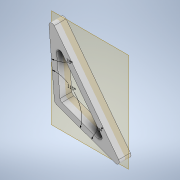
# Autodesk Inventor part: stopForSaltChute
Saved by Autodesk Inventor 2021.1 (Build 251245000, 245)
## iProperties
Created: 2020-09-07
Part Number: stopForSaltChute
Material: Generic
Document SubType Name: Modeling
Designer: robst
Density: 1 g/cm^3
Appearance: Default
Author: robst
Autodesk Inventor part; units mm, degrees
ref_plane "YZ Plane" through (0, 0, 0) normal (1, 0, 0) x (0, 1, 0)
ref_plane "XZ Plane" through (0, 0, 0) normal (0, 1, 0) x (-1, 0, 0)
sketch "Sketch1" plane through (0, 0, 0) normal (0, 0, 1) x (1, 0, 0)
  line L0 (0, 0) -> (-10.4993, 120.0076)
  line L1 (-10.4993, 120.0076) -> (113.201, -41.2018)
  line L2 (113.201, -41.2018) -> (0, 0)
  dimension "d23" = 115
  dimension "d24" = 203.2
  dimension "d31" = 32.5
  constraints: 6 end point
  measures "d23" angle of L2 L0
  measures "d24" distance of L0.end L1.end
  measures "d31" angle of L1 L2
extrude "Extrusion1" add sketch "Sketch1" along normal mid plane 19.05
sketch "Sketch2" plane through (0, 0, 0) normal (0, 0, 1) x (1, 0, 0)
  line L0 (8.9599, 6.8752) -> (1.8376, 88.2833)
  line L1 (1.8376, 88.2833) -> (85.7507, -21.0744)
  line L2 (85.7507, -21.0744) -> (8.9599, 6.8752)
  line L3 (0, 0) -> (-10.4993, 120.0076) projected
  line L4 (-10.4993, 120.0076) -> (113.201, -41.2018) projected
  line L5 (113.201, -41.2018) -> (0, 0) projected
  dimension "d4" = 9.525
  dimension "d5" = 9.525
  dimension "d6" = 9.525
  constraints: 6 end point, 3 parallel, 1 equal length, 1 other
  measures "d4" distance between parallel lines of L0 L3
  measures "d5" distance between parallel lines of L1 L4
  measures "d6" distance between parallel lines of L2 L5
extrude "Extrusion2" cut sketch "Sketch2" against normal through all both and the other way through all contours L0 L1 L2
fillet "Fillet1" radius 4.7625 3 edges at (-10.4993, 120.0076, 0) (0, 0, 0) (113.201, -41.2018, 0)
fillet "Fillet2" radius 4.7625 3 edges at (1.8376, 88.2833, 0) (8.9599, 6.8752, 0) (85.7507, -21.0744, 0)
equation "\"d23\" = longAngle"
equation "\"d24\" = maxLength"
equation "\"d31\" = basicAngle"
equation "\"d2\" = width"
equation "\"d4\" = wallThickness"
equation "\"d5\" = wallThickness"
equation "\"d6\" = wallThickness"
equation "\"d32\" = fillet"
equation "\"d33\" = fillet"
equation "\"maxLength\" = 203.2"
equation "\"width\" = 19.05"
equation "\"wallThickness\" = 9.525"
equation "\"longAngle\" = 115deg"
equation "\"fillet\" = 4.7625"
equation "\"basicAngle\" = 32.5deg"
body "Solid1"
